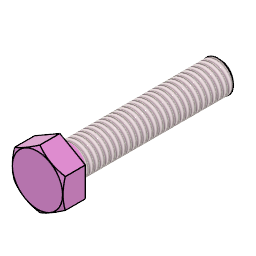
lamp (Autodesk Fusion 360 archive; units mm, degrees)
design "Hex Head Bolt JIS B 1180 - M3x15 - C Steel 4.6 Plain"
description: Hex Head Bolt JIS B 1180 - M3x15 - C
part number: JIS B 1180 - M3x15 C Steel 4.6 Plain
Autodesk Fusion 360 part; units mm, degrees
sketch "Sketch1" plane through (0, 0, 0) normal (0, 1, 0) x (1, 0, 0)
  line L0 (-1.5, 0) -> (-1.5, 15)
  line L1 (-1.5, 15) -> (0, 15)
  line L2 (0, 15) -> (0, -2.1)
  line L3 (-1.5, 0) -> (-2.7427, 0)
  line L4 (-2.7427, 0) -> (-2.7427, -1.8744)
  line L5 (-2.352, -2.1) -> (0, -2.1)
  line L6 (-2.7427, -1.8744) -> (-2.352, -2.1)
  dimension "d81" = 5.4854
  dimension "d135" = 3
  dimension "d139" = 2.1
  dimension "d140" = 15
  dimension "d156" = 4.704
  dimension "d158" = 30
  constraint perpendicular L0 L1
  constraint collinear origin L1.end L2.end
  constraint perpendicular L0 L3
  constraint coincident origin L3
  constraint vertical L2
  constraint coincident L2 L5.end
  constraint coincident L0.start L3.start
  constraint coincident L0.end L1.start
  constraint vertical L4
  measures "d139" distance of L3 L5
  measures "d140" distance of L1 L3
  measures "d158" angle of L5 L6
revolve "Revolve1" add sketch "Sketch1" angle 360 about axis through (0, 0, -15) along (0, 0, 1)
sketch "Sketch8" plane through (0, 0, 2.1) normal (0, 0, 1) x (1, 0, 0)
  circle A0 centre (0, 0) radius 2.7427
  line L0 (-2.3753, -1.3714) -> (0, -2.7427)
  line L1 (0, -2.7427) -> (2.3753, -1.3714)
  line L2 (2.3753, -1.3714) -> (2.3753, 1.3714)
  line L3 (2.3753, 1.3714) -> (0, 2.7427)
  line L4 (0, 2.7427) -> (-2.3753, 1.3714)
  line L5 (-2.3753, 1.3714) -> (-2.3753, -1.3714)
  constraint coincident A0 L0.start
  constraint coincident A0.centre origin
  constraint vertical L5
extrude "Extrude5" cut sketch "Sketch8" against normal blind 2.1 contours A0 L2 | A0 L3 | A0 L1 | A0 L4 | A0 L0 | A0 L5
fillet "Fillet7" radius 0.12 1 edges at (-1.3985, 0.5424, 0)
thread "Thread4" "ISO Metric profile 3.0 M3x0.5 M3x0.5 6g" major diameter 2.927 minor diameter 2.3555 pitch 0.5 angle 60 resizes the face on face at (-1.4981, 0.0748, -5.08) from (0, 0, -1) to (0, 0, -15)
sketch "Sketch13" plane through (0, 0, 0) normal (0, 1, 0) x (1, 0, 0)
  line L0 (0, 15) -> (0, -2.1) construction
  line L1 (0, 15) -> (-1.53, 15)
  line L2 (-1.53, 15) -> (-1.53, 14.7)
  line L3 (-1.53, 14.7) -> (-1.2, 15)
  dimension "d160" = 0.3
  dimension "d161" = 1.2
  dimension "d162" = 1.53
  constraint coincident L0.start L1.start
  constraint perpendicular L0 L1
  constraint perpendicular L1 L2
  constraint coincident L1 L3.end
  measures "d160" distance of L1 L2.end
  measures "d161" distance of L0 L3.end
  measures "d162" distance of L0.start L2
revolve "Revolve4" cut sketch "Sketch13" angle 360 about axis through (0, 0, 1.75) along (0, 0, 1)
equation "adsk_nomlen = 15.00 mm"
equation "adsk_headh = 2.10 mm"
equation "adsk_headdia = 5.48544 mm"
equation "adsk_nomdia = 3.00 mm"
equation "d81 = adsk_headdia"
equation "d89 = -adsk_headh"
equation "adsk_waflat = 4.80 mm"
equation "adsk_thrlen = 14.00 mm"
equation "adsk_midfillet = 0.12 mm"
equation "d135 = adsk_nomdia"
equation "d139 = adsk_headh"
equation "d140 = adsk_nomlen"
equation "d142 = adsk_midfillet"
equation "adsk_endpointdia = adsk_nomdia - adsk_startlen * 2"
equation "adsk_startlen = 0.1 * adsk_nomdia"
equation "d156 = adsk_waflat * 0.98"
equation "d158 = adsk_chamang2"
equation "adsk_chamang2 = 30.00 deg"
equation "d160 = adsk_startlen"
equation "d161 = adsk_endpointdia / 2"
equation "d162 = adsk_nomdia * 0.51"
equation "d166 = min(adsk_thrlen; adsk_nomlen - adsk_midfillet - 0.001 mm)"

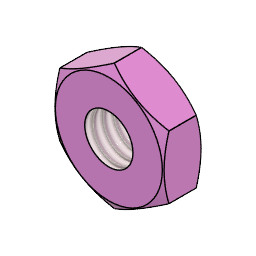
design "Chamfered Bottom Hex Machine Screw Nut ANSI B18.6.3 - 3-56 Steel Grade 2H Plain"
description: Chamfered Bottom Hex Machine Screw Nut ANSI B18.6.3 - 3-56
part number: CBHMSN ANSI B18.6.3 - 3-56 Steel Grade 2H Plain
Autodesk Fusion 360 part; units mm, degrees
sketch "Sketch1" plane through (0, 0, 0) normal (0, 1, 0) x (1, 0, 0)
  line L0 (0, 0) -> (0, -1.6764)
  line L1 (-1.2573, 0) -> (-2.3398, 0)
  line L2 (-2.3398, 0) -> (-2.7559, -0.2402)
  line L3 (-2.7559, -0.2402) -> (-2.7559, -1.4362)
  line L4 (-2.7559, -1.4362) -> (-2.3398, -1.6764)
  line L5 (-2.3398, -1.6764) -> (-1.2573, -1.6764)
  line L6 (-1.2573, -1.6764) -> (-1.2573, 0)
  dimension "d121" = 2.5146
  dimension "d122" = 30
  dimension "d123" = 30
  dimension "d128" = 5.5118
  dimension "d142" = 4.6797
  dimension "d146" = 1.6764
  constraint vertical L0
  constraint coincident L0 L0.end
  constraint coincident origin L0
  constraint horizontal L1
  constraint coincident L0.start L1
  constraint coincident L0.start origin
  constraint vertical L1.end L4.end
  constraint coincident L0.end L5
  measures "d122" angle of L1 L2
  measures "d123" angle of L4 L5
  measures "d146" distance of L1 L5
revolve "Revolve1" add sketch "Sketch1" angle 360 about axis through (0, 0, 0) along (0, 0, 1)
sketch "Sketch8" plane through (0, 0, 1.6764) normal (0, 0, 1) x (1, 0, 0)
  line L0 (-2.3876, -1.3764) -> (-2.3876, 1.3764)
  circle A0 centre (0, 0) radius 1.2573
  circle A1 centre (0, 0) radius 2.7559
  dimension "d114" = 2.3876
  constraint coincident L0.end A1
  constraint coincident L0.start A1
  constraint vertical L0
  measures "d114" distance of A0.centre L0
extrude "Extrude5" cut sketch "Sketch8" against normal blind 1.6764 contours L0 A1 picked at (-2.447, -0.3352)
pattern_circular "C-Pattern2" count 6 over 360 about axis through (0, 0, 1.75) along (0, 0, 1) of "Extrude5"
thread "Thread3" "ANSI Unified Screw Threads 0.099(#3) 3-56 UNF 3-56 UNF 2B" major diameter 2.5146 minor diameter 2.1107 pitch 0.4536 angle 60 resizes the face on face at (-1.2557, 0.0627, 1.1176)
equation "d89 = -adsk_nheig"
equation "d114 = adsk_waflat / 2"
equation "adsk_chamang1 = 30 deg"
equation "adsk_chamang2 = 30 deg"
equation "d121 = adsk_nomdia"
equation "d122 = adsk_chamang1"
equation "d123 = adsk_chamang2"
equation "d128 = adsk_maxdia"
equation "adsk_nheig = 0.066 in"
equation "adsk_maxdia = 0.217 in"
equation "adsk_nomdia = 0.099 in"
equation "adsk_waflat = 0.188 in"
equation "d139 = adsk_nheig"
equation "adsk_beardia = adsk_waflat * 0.98"
equation "d142 = adsk_beardia"
equation "d146 = adsk_nheig"
